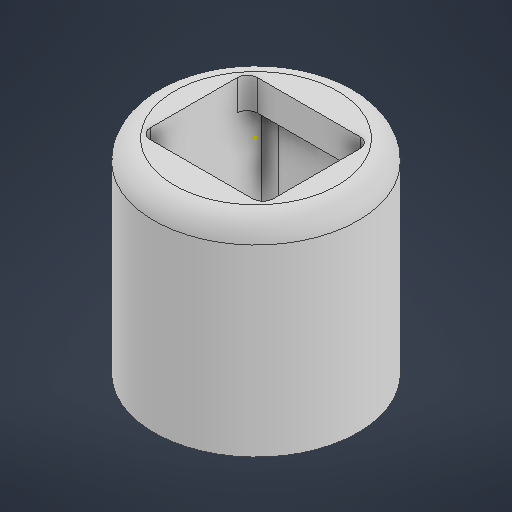
# Autodesk Inventor part: module
Saved by Autodesk Inventor 2026.2 (Build 302298000, 298)
## iProperties
Created: 2026-01-25
Part Number: module
Material: Generic
Document SubType Name: Modeling
Designer: Koda
Density: 1 g/cm^3
Appearance: Default
Author: Koda
Autodesk Inventor part; units mm, degrees
ref_plane "YZ Plane" through (0, 0, 0) normal (1, 0, 0) x (0, 1, 0)
ref_plane "XZ Plane" through (0, 0, 0) normal (0, 1, 0) x (-1, 0, 0)
ref_plane "XY Plane" through (0, 0, 0) normal (0, 0, 1) x (1, 0, 0)
sketch "Sketch1" plane through (0, 0, 0) normal (0, 1, 0) x (-1, 0, 0)
  circle A0 centre (0, 0) radius 15.875
  dimension "d0" = 31.75
  constraints: 1 centre point, 1 coincident
  measures "d0" diameter of A0
extrude "Extrusion1" add sketch "Sketch1" along normal blind 31.75
fillet "Fillet1" radius 3.175 1 edges at (15.875, 31.75, 0)
sketch "Sketch2" plane through (0, 31.75, 0) normal (0, 1, 0) x (1, 0, 0)
  point P0 (0, 0)
sketch "Sketch3" plane through (0, 0, 0) normal (0, -1, 0) x (1, 0, 0)
  circle A0 centre (0, 0) radius 12.7
  line L0 (-7.091, -10.536) -> (-9.6294, -10.536)
  line L1 (-9.6294, -10.536) -> (-9.6294, 8.2804)
  line L2 (-9.6294, 8.2804) -> (-7.091, 8.2804)
  line L3 (-7.091, 8.2804) -> (-7.091, -10.536)
  line L4 (-7.091, 10.536) -> (-9.6294, 10.536)
  line L5 (-9.6294, 10.536) -> (-9.6294, 8.2804)
  line L6 (-9.6294, 8.2804) -> (-7.091, 8.2804)
  line L7 (-7.091, 8.2804) -> (-7.091, 10.536)
  constraints: 16 end point, 4 parallel, 3 point on circle, 2 horizontal, 2 perpendicular, 1 centre point, 1 coincident, 1 point on line
extrude "Extrusion2" cut sketch "Sketch3" against normal blind 26.9875 contours A0 L3 L7 | L7 L2 A0 | A0 L5 L4 | L0 L1 A0 | A0 L1 L2 L3
sketch "Sketch4" plane through (0, 31.75, 0) normal (0, 1, 0) x (1, 0, 0)
  circle A0 centre (0, 0) radius 12.7
  line L0 (-9.6294, 10.536) -> (-9.6294, -10.536) projected
  line L1 (-9.6294, 8.2804) -> (9.5066, 8.2804)
  line L2 (9.5066, 8.2804) -> (9.5066, -8.4211)
  line L3 (9.5066, -8.4211) -> (-9.6294, -8.4211)
  line L4 (-9.6294, -8.4211) -> (-9.6294, 8.2804)
  point P0 (-9.5066, -8.4211)
  point P1 (-9.6294, -8.2804)
  constraints: 8 end point, 2 parallel, 2 point on circle, 1 centre point, 1 coincident, 1 horizontal, 1 perpendicular, 1 point on line
extrude "Extrusion3" cut sketch "Sketch4" against normal blind 4.7625 contours L1 L2 L3 A0 L0
fillet "Fillet2" radius 1.5875 5 edges at (-9.6294, 29.3687, -8.2804) (9.5066, 29.3687, -8.2804) (9.5066, 29.3687, 8.4211) (-9.6294, 29.3687, 8.2804) (-9.5066, 29.3687, 8.4211)
sketch "Sketch5" plane through (-9.6294, 0, 10.536) normal (1, 0, 0) x (0, 0, -1)
  circle A0 centre (10.536, 2.4407) radius 2
  point P0 (10.536, 0)
  dimension "d9" = 4
  constraints: 1 centre point
  measures "d9" diameter of A0
extrude "Extrusion4" cut sketch "Sketch5" against normal blind 5
body "Solid1"
